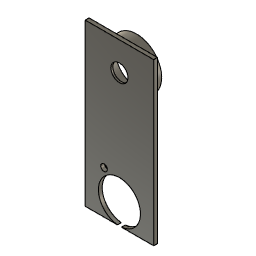
Robotic_Arm_Initial_Design v1 (Autodesk Fusion 360 archive; units mm, degrees)
design "Trial_6"
Autodesk Fusion 360 part; units mm, degrees
sketch "Sketch1" plane through (0, 0, 0) normal (0, 1, 0) x (1, 0, 0)
  line L0 (0, 0) -> (36, 0)
  line L1 (36, 0) -> (36, -69.7)
  line L2 (36, -69.7) -> (0, -69.7)
  line L3 (0, -69.7) -> (0, 0)
  dimension "d1" = 36
  dimension "d2" = 69.7
  constraint horizontal L0
  constraint vertical L1
  constraint horizontal L2
  constraint vertical L3
  constraint coincident L0.start L3.end
  measures "d1" distance of L0.start L0.end
  measures "d2" distance of L0.start L2.end
sketch "Sketch2" plane through (0, 0, 0) normal (0, 1, 0) x (1, 0, 0)
  line L0 (0, 0) -> (18, 0)
  line L1 (18, 0) -> (18, -11)
  circle A0 centre (18, -11) radius 11.05
  line L2 (18, -11) -> (18, -69.7)
  circle A1 centre (18, -69.7) radius 11.2
  circle A2 centre (18, -69.7) radius 4.5
  line L3 (-0.000001, -81.7) -> (36, -81.7)
  line L4 (36, -81.7) -> (36, -69.7)
  line L5 (36, -69.7) -> (-0.000001, -69.7)
  line L6 (-0.000001, -69.7) -> (-0.000001, -81.7)
  circle A3 centre (18, -11) radius 14.05
  circle A4 centre (9.924693, -22.497475) radius 1.75
  circle A5 centre (18, -69.7) radius 13.2
  line L7 (36, -81.7) -> (0, -81.7)
  line L8 (0, -81.7) -> (0, -84.7)
  line L9 (0, -84.7) -> (36, -84.7)
  line L10 (36, -84.7) -> (36, -81.7)
  point P0 (36, -69.7)
  dimension "d3" = 18
  dimension "d4" = 11
  dimension "d5" = 22.1
  dimension "d6" = 58.7
  dimension "d7" = 22.4
  dimension "d8" = 9
  dimension "d9" = 28.1
  dimension "d10" = 3.5
  dimension "d11" = 2
  dimension "d28" = 3
  constraint coincident L0.start origin
  constraint horizontal L0
  constraint perpendicular L0 L1
  constraint coincident L1.end A0.centre
  constraint parallel L1 L2
  constraint coincident L2.end A1.centre
  constraint concentric A1 A2
  constraint horizontal L3
  constraint vertical L4
  constraint horizontal L5
  constraint vertical L6
  constraint coincident P0 L4.end
  constraint concentric A0 A3
  constraint horizontal L7
  constraint vertical L8
  constraint horizontal L9
  constraint vertical L10
  measures "d3" distance of L0.start L0.end
  measures "d4" distance of L0.end L1.end
  measures "d5" diameter of A0
  measures "d6" distance of L1.end L2.end
  measures "d7" diameter of A1
  measures "d8" diameter of A2
  measures "d9" diameter of A3
  measures "d10" diameter of A4
  measures "d28" distance of L3.end L9.end
extrude "Extrude1" add sketch "Sketch2" sketch "Sketch1" along normal blind 2 contours A1 L3 L5 A5 L7 | L3 L4 L5 A5 L7 | L3 L5 L6 A5 L7 | A1 A2 L5 | A2 L5 picked at (24.082727, -80.631967) picked at (34.222172, -74.93825) picked at (1.777828, -74.93825) picked at (9.091785, -70.479988) picked at (20.983246, -69.923563) of sketch 2 contours L0 L1 L2 L3 picked at (12, -23.233333)
sketch "Sketch3" plane through (0, 2, 0) normal (0, 1, 0) x (-1, 0, 0)
  line L0 (0, 0) -> (0.000001, 81.7)
  line L1 (0.000001, 81.7) -> (-36, 81.7)
  line L2 (-36, 81.7) -> (-36, 0)
  line L3 (-36, 0) -> (0, 0)
  circle A0 centre (-18, 69.699998) radius 11.2
  circle A1 centre (-18, 69.699998) radius 13.2
  line L4 (-36, 81.7) -> (0, 81.7)
  line L5 (0, 81.7) -> (0, 84.7)
  line L6 (0, 84.7) -> (-36, 84.7)
  line L7 (-36, 84.7) -> (-36, 81.7)
  dimension "d14" = 22.4
  dimension "d15" = 2
  dimension "d29" = 3
  constraint horizontal L4
  constraint vertical L5
  constraint horizontal L6
  constraint vertical L7
  constraint coincident L1.end L2.start
  measures "d14" diameter of A0
  measures "d29" distance of L1.end L6.end
extrude "Extrude2" add sketch "Sketch3" along normal blind 7 contours L1 A1 L4 | L1 A1 L4 picked at (-24.101343, 80.619905) picked at (-19.243282, 81.920692)
extrude "Extrude3" cut sketch "Sketch2" along normal blind 3.5 contours L2 A2 L5 | L2 A2 L5 | A2 L5 picked at (20.803687, -68.654279) picked at (15.015268, -69.486528) picked at (20.983246, -69.923563)
extrude "Extrude4" cut sketch "Sketch2" along normal blind 16 contours L0 L1 A0 L2 | L0 L1 A0 L2 picked at (18.668462, -3.711165) picked at (17.467539, -18.327977)
extrude "Extrude5" cut sketch "Sketch2" along normal blind 12.5 contours A3 A4 | A3 A4 picked at (10.236715, -21.995081) picked at (9.594065, -22.968217)
extrude "Extrude6" cut sketch "Sketch2" along normal blind 40 contours L2 A1 A2 L5 | L2 A1 A2 L5 | A1 A2 L5 picked at (26.71668, -67.694291) picked at (9.28332, -67.694291) picked at (9.091785, -70.479988)
sketch "Sketch4" plane through (0, 0, 0) normal (0, -1, 0) x (1, 0, 0)
  circle A0 centre (18, 69.7) radius 11.2
  circle A1 centre (9.924693, 22.497475) radius 1.75
  arc A2 (19.05, 0) -> (16.95, 0) centre (18, 11) ccw
  line L0 (19.05, 0) -> (36, 0)
  line L1 (36, 0) -> (36, 81.7)
  line L2 (36, 81.7) -> (-0.000001, 81.7)
  line L3 (-0.000001, 81.7) -> (0, 0)
  line L4 (0, 0) -> (16.95, 0)
sketch "Sketch5" plane through (0, 9, 0) normal (0, 1, 0) x (-1, 0, 0)
  circle A0 centre (-18, 69.699998) radius 11.2
  circle A1 centre (-18, 69.699998) radius 13.2
extrude "Extrude7" add sketch "Sketch2" along normal blind 1 contours L2 A1 A2 L5 | L2 A1 A2 L5 | A1 A2 L5 picked at (26.71668, -67.694291) picked at (9.28332, -67.694291) picked at (9.091785, -70.479988)
delete_face "DeleteFace1" 1 faces at (18, 6.666667, 82.899998)
extrude "Extrude8" add sketch "Sketch3" against normal blind 2 contours L1 A1 L4 L5 L6 L7 | L1 A1 L4 picked at (-4.166971, 82.7) picked at (-19.243282, 81.920692)
extrude "Extrude9" add sketch "Sketch3" along normal blind 7 contours L1 A1 L4 | L1 A1 L4 picked at (-24.101343, 80.619905) picked at (-19.243282, 81.920692)
